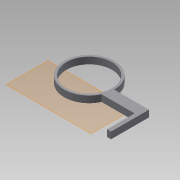
# Autodesk Inventor part: 16_Gabel
Saved by Autodesk Inventor 2015 (Build 190159000, 159)
## iProperties
Created: 2016-03-16
Part Number: 16_Gabel
Material: Generisch
Document SubType Name: Modeling
Designer: Bene
Density: 1 g/cm^3
Appearance: Vorgabe
Author: Bene
Autodesk Inventor part; units mm, degrees
ref_plane "YZ Plane" through (0, 0, 0) normal (1, 0, 0) x (0, 1, 0)
ref_plane "XZ Plane" through (0, 0, 0) normal (0, 1, 0) x (-1, 0, 0)
ref_plane "Arbeitsebene1" through (0, 0, 0) normal (0, 0, 1) x (1, 0, 0)
sketch "Skizze1" plane through (0, 0, 0) normal (0, 0, 1) x (1, 0, 0)
  circle A0 centre (-1.9028, 0) radius 18.75 projected
  circle A1 centre (-1.9028, 0) radius 16.25 projected
  line L0 (31.75, -9) -> (39.5, -9) projected
  line L1 (39.5, -9) -> (39.5, -29) projected
  circle A2 centre (-1.9028, 0) radius 17.0624
  line L2 (39.9814, -7.7741) -> (15.1596, -7.7741)
  line L3 (15.1596, -7.7741) -> (15.1596, 0)
  line L4 (15.1596, 0) -> (39.9814, 0)
  line L5 (39.9814, 0) -> (39.9814, -7.7741)
  line L6 (39.9814, 0) -> (42.9814, 0)
  line L7 (42.9814, 0) -> (42.9814, -28.4525)
  line L8 (42.9814, -28.4525) -> (39.9814, -28.4525)
  line L9 (39.9814, -28.4525) -> (39.9814, 0)
  point P0 (0, 0)
  dimension "d0" = 3
  constraints: 16 end point, 4 parallel, 2 horizontal, 2 perpendicular, 1 horizontal alignment, 4 other
  measures "d0" distance of L7.end L8.end
extrude "Extrusion1" add sketch "Skizze1" along normal blind 5 contours L4 L3 A0 | L4 L5 L2 A0 | A0 L3 L4 | L6 L7 L8 L9 L5
sketch "Skizze2" plane through (0, 0, 5) normal (0, 0, 1) x (1, 0, 0)
  arc A0 (16.8472, 0) -> (15.1596, -7.7741) centre (-1.9028, 0) ccw projected
  line L0 (15.1596, -7.7741) -> (39.9814, -7.7741) projected
  line L1 (39.9814, -7.7741) -> (39.9814, -28.4525) projected
  line L2 (39.9814, -28.4525) -> (42.9814, -28.4525) projected
  line L3 (42.9814, -28.4525) -> (42.9814, 0) projected
  line L4 (42.9814, 0) -> (16.8472, 0) projected
  circle A1 centre (-1.9028, 0) radius 17.0624 projected
  line L5 (42.9814, 0) -> (39.9814, 0)
  line L6 (39.9814, 0) -> (39.9814, -28.4525)
  line L7 (39.9814, -28.4525) -> (42.9814, -28.4525)
  line L8 (42.9814, -28.4525) -> (42.9814, 0)
  point P0 (0, 0)
  constraints: 8 end point, 2 parallel, 1 horizontal, 1 perpendicular
ref_plane "Arbeitsebene2" through (31.75, -29, 35) normal (0, 0, 1) x (1, 0, 0)
extrude "Extrusion2" add sketch "Skizze2" along normal up to surface (30 mm away) contours L4 L3 L2 L1 L6
sketch "Skizze3" plane through (42.9814, -28.4525, 0) normal (1, 0, 0) x (0, 0, -1)
  line L0 (-35, 13.9525) -> (6, 13.9525) projected
  line L1 (-35, 13.9525) -> (6, 13.9525) projected
  circle A0 centre (-6, 16.9525) radius 1.5 projected
  circle A1 centre (-23, 16.9525) radius 1.5 projected
  circle A2 centre (-6, 2.2025) radius 1.5 projected
  circle A3 centre (-23, 1.9525) radius 1.5 projected
  circle A4 centre (-23, 25.4997) radius 1.5
  circle A5 centre (-7.5, 25.4997) radius 1.5
  point P0 (0, 28.4525)
  dimension "d7" = 3
  dimension "d8" = 3
  constraints: 2 centre point
  measures "d7" diameter of A4
  measures "d8" diameter of A5
extrude "Extrusion3" cut sketch "Skizze3" against normal blind 5
